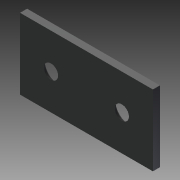
# Autodesk Inventor part: MGCE1plate5-5
Saved by Autodesk Inventor 2011 SP1 (Build 150282100, 282)
## iProperties
Created: 2015-02-01
Part Number: MGCE1plate5-5
Catalog Web Link: www.cadenas.de
Description: MGCE1plate-MAgnet Catches for Frames - Magnet Plate
Vendor: MISUMI
Document SubType Name: Modeling
Designer: PARTuser1
Manufacturer: MISUMI
Mass: 0.708146 g
Surface Area: 10.9727 cm^2
Volume: 0.708146 cm^3
Density: 1 g/cm^3
Category: PARTsolutions
Company: MISUMI
Title: MGCE1plate5-5
Author: Cadenas PARTsolutions
Comments: MAgnet Catches for Frames - Magnet Plate
PSOL_IDENT_0: {\\10.0.0.236\data_v8\23d-libs\misumi\metric\39_accessories_for_al_extrusions\hmgce_mgplate.prj},172
PSOL_IDENT_1: {VTYP=3D},{NB=MGCE1plate5-5},{LINA=MGCE1plate5-5},{NN=MGCE1plate},{DATE=17.11.2014 05:31:13},{GEOMD
PSOL_IDENT_2: ATE=28.07.2009 05:42:00},{VERSION=},{LINEID=10},{LINESUBID=-1},{WBVAR=}  {NB=MGCE1plate5-5},{LINA=MG
PSOL_IDENT_3: CE1plate5-5},{KT=DUMMY},{PN=MGCE1plate5-5},{TYPE=MGCE1plate},{NO=5-5}
SUPPLIER: MISUMI
ARTICLENO: MGCE1plate5-5
BOMINFO: MGCE1plate5-5
CREATOR: CADENAS GmbH
Autodesk Inventor part; units mm, degrees
sketch "Sketch_1" plane through (0, 0, 0) normal (0, 0, 1) x (1, 0, 0)
  line L0 (-15, 0) -> (15, 0)
  line L1 (15, 0) -> (15, 1.6)
  line L2 (15, 1.6) -> (-15, 1.6)
  line L3 (-15, 1.6) -> (-15, 0)
  constraints: 8 end point
extrude "Extrusion1" add sketch "Sketch_1" along normal mid plane 16
sketch "Sketch_2" plane through (0, 0, 0) normal (0, 0, 1) x (1, 0, 0)
  line L0 (8, 0) -> (8, 1.6)
  line L1 (8, 1.6) -> (11.1, 1.6)
  line L2 (11.1, 1.6) -> (11.1, 1.5)
  line L3 (11.1, 1.5) -> (9.6, 0)
  line L4 (9.6, 0) -> (8, 0)
  line L5 (8, 0) -> (8, 1.6)
  constraints: 12 end point
revolve "Revolution1" cut sketch "Sketch_2" angle 360 about axis through (8, 0, 0) along (0, -1, 0)
sketch "Sketch_3" plane through (0, 0, 0) normal (0, 0, 1) x (1, 0, 0)
  line L0 (-8, 0) -> (-8, 1.6)
  line L1 (-8, 1.6) -> (-4.9, 1.6)
  line L2 (-4.9, 1.6) -> (-4.9, 1.5)
  line L3 (-4.9, 1.5) -> (-6.4, 0)
  line L4 (-6.4, 0) -> (-8, 0)
  line L5 (-8, 0) -> (-8, 1.6)
  constraints: 12 end point
revolve "Revolution2" cut sketch "Sketch_3" angle 360 about axis through (-8, 0, 0) along (0, -1, 0)
ref_plane "to_magnet_XY" through (0, 1.6, 0) normal (0, -1, 0) x (1, 0, 0)
ref_plane "to_magnet_YZ" through (0, 1.6, 0) normal (1, 0, 0) x (0, 0, 1)
ref_plane "to_magnet_ZX" through (0, 1.6, 0) normal (0, 0, 1) x (0, -1, 0)
ref_plane "to_bolt1_XY" through (-8, 0.1, 0) normal (0, 1, 0) x (1, 0, 0)
ref_plane "to_bolt1_YZ" through (-8, 0.1, 0) normal (1, 0, 0) x (0, 0, -1)
ref_plane "to_bolt1_ZX" through (-8, 0.1, 0) normal (0, 0, -1) x (0, 1, 0)
ref_plane "to_bolt2_XY" through (8, 0.1, 0) normal (0, 1, 0) x (1, 0, 0)
ref_plane "to_bolt2_YZ" through (8, 0.1, 0) normal (1, 0, 0) x (0, 0, -1)
ref_plane "to_bolt2_ZX" through (8, 0.1, 0) normal (0, 0, -1) x (0, 1, 0)
body "Solid1"
